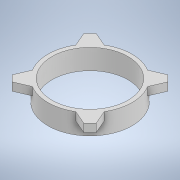
# Autodesk Inventor part: FläktHållare
Saved by Autodesk Inventor 2021 (Build 250183000, 183)
## iProperties
Created: 2025-01-14
Part Number: FläktHållare
Material: Generic
Document SubType Name: Modeling
Designer: 24lucsil
Density: 1 g/cm^3
Appearance: Default
Author: 24lucsil
Autodesk Inventor part; units mm, degrees
ref_plane "YZ Plane" through (0, 0, 0) normal (1, 0, 0) x (0, 1, 0)
ref_plane "XZ Plane" through (0, 0, 0) normal (0, 1, 0) x (-1, 0, 0)
ref_plane "XY Plane" through (0, 0, 0) normal (0, 0, 1) x (1, 0, 0)
sketch "Sketch1" plane through (0, 0, 0) normal (0, 1, 0) x (-1, 0, 0)
  circle A0 centre (0, 0) radius 47
  circle A1 centre (0, 0) radius 52
  line L0 (52, -52) -> (-52, -52) construction
  line L1 (-52, -52) -> (-52, 52) construction
  line L2 (-52, 52) -> (52, 52) construction
  line L3 (52, 52) -> (52, -52) construction
  line L4 (52, -52) -> (52, -44.5) construction
  line L5 (52, -52) -> (44.5, -52) construction
  line L6 (-52, -52) -> (-44.5, -52) construction
  line L7 (-52, -52) -> (-52, -44.5) construction
  line L8 (-52, 52) -> (-44.5, 52) construction
  line L9 (-52, 52) -> (-52, 44.5) construction
  line L10 (52, 52) -> (52, 44.5) construction
  line L11 (52, 52) -> (44.5, 52) construction
  line L12 (52, 52) -> (52, 44.5) construction
  line L13 (52, -44.5) -> (44.5, -52)
  line L14 (-44.5, -52) -> (-52, -44.5)
  line L15 (-52, 44.5) -> (-44.5, 52)
  line L16 (44.5, 52) -> (52, 44.5)
  line L17 (44.5, -52) -> (44.5, -26.9026) construction
  line L18 (52, -44.5) -> (44.5, -26.9026) construction
  line L19 (-44.5, -52) -> (-44.5, -26.9026) construction
  line L20 (-52, -44.5) -> (-44.5, -26.9026) construction
  line L21 (52, -44.5) -> (26.9026, -44.5) construction
  line L22 (44.5, -52) -> (26.9026, -44.5) construction
  line L23 (-52, -44.5) -> (-26.9026, -44.5) construction
  line L24 (-44.5, -52) -> (-26.9026, -44.5) construction
  line L25 (-44.5, 52) -> (-44.5, 26.9026) construction
  line L26 (-52, 44.5) -> (-44.5, 26.9026) construction
  line L27 (-52, 44.5) -> (-26.9026, 44.5) construction
  line L28 (-44.5, 52) -> (-26.9026, 44.5) construction
  line L29 (52, 44.5) -> (26.9026, 44.5) construction
  line L30 (44.5, 52) -> (44.5, 26.9026) construction
  line L31 (44.5, 52) -> (26.9026, 44.5) construction
  line L32 (52, 44.5) -> (44.5, 26.9026) construction
  line L33 (44.5, 52) -> (26.9026, 44.5)
  line L34 (52, 44.5) -> (44.5, 26.9026)
  line L35 (52, -44.5) -> (44.5, -26.9026)
  line L36 (44.5, -52) -> (26.9026, -44.5)
  line L37 (-26.9026, -44.5) -> (-44.5, -52)
  line L38 (-44.5, -26.9026) -> (-52, -44.5)
  line L39 (-44.5, 26.9026) -> (-52, 44.5)
  line L40 (-44.5, 52) -> (-26.9026, 44.5)
  dimension "d1" = 104
  dimension "d0" = 94
  dimension "d6" = 7.5
  dimension "d7" = 7.5
  dimension "d8" = 7.5
  dimension "d9" = 7.5
  dimension "d10" = 7.5
  dimension "d11" = 7.5
  dimension "d12" = 104
  dimension "d13" = 104
  dimension "d15" = 7.5
  dimension "d16" = 7.5
  dimension "d18" = 96.5
  constraints: 82 end point, 10 point on line, 9 perpendicular, 2 coincident, 2 horizontal, 2 vertical, 1 centre point, 1 collinear, 10 other
  measures "d0" diameter of A0
  measures "d6" distance of L0.start L4.end
  measures "d7" distance of L0.start L5.end
  measures "d8" distance of L0.end L6.end
  measures "d9" distance of L9.end L1.end
  measures "d10" distance of L1.end L8.end
  measures "d11" distance of L0.end L7.end
  measures "d12" distance of L1.end L2.end
  measures "d13" distance of L2.end L0.start
  measures "d15" distance from line of L11.end L3
  measures "d16" distance of L10.end L2.end
  measures "d18" distance from line of L37.end L12
extrude "Extrusion1" add sketch "Sketch1" along normal blind 25 contours A1
sketch "Sketch2" plane through (0, 25, 0) normal (0, 1, 0) x (1, 0, 0)
  line L0 (-52, -52) -> (-52, 52) construction
  line L1 (-52, 52) -> (52, 52) construction
  line L2 (52, 52) -> (52, -52) construction
  line L3 (52, -52) -> (-52, -52) construction
  line L4 (-52, -52) -> (-44.5, -52) construction
  line L5 (52, -52) -> (44.5, -52) construction
  line L6 (52, -52) -> (52, -44.5) construction
  line L7 (52, 52) -> (52, 44.5) construction
  line L8 (-52, 52) -> (-52, 44.5) construction
  line L9 (-52, 52) -> (-44.5, 52) construction
  line L10 (52, 52) -> (44.5, 52) construction
  line L11 (52, 44.5) -> (44.5, 52)
  line L12 (-44.5, 52) -> (-52, 44.5)
  line L13 (-44.5, -52) -> (-52, -44.5)
  line L14 (44.5, -52) -> (52, -44.5)
  circle A0 centre (0, 0) radius 52 construction
  line L15 (-52, 44.5) -> (-44.5, 26.9026)
  circle A1 centre (0, 0) radius 52 projected
  line L16 (52, 44.5) -> (44.5, 26.9026)
  line L17 (-44.5, 52) -> (-26.9026, 44.5)
  line L18 (44.5, 52) -> (26.9026, 44.5)
  line L19 (52, -44.5) -> (44.5, -26.9026)
  line L20 (44.5, -52) -> (26.9026, -44.5)
  line L21 (-44.5, -52) -> (-26.9026, -44.5)
  line L22 (-52, -44.5) -> (-44.5, -26.9026)
  dimension "d19" = 104
  dimension "d20" = 104
  dimension "d21" = 52
  dimension "d22" = 52
  dimension "d23" = 7.5
  dimension "d24" = 7.5
  dimension "d25" = 7.5
  dimension "d26" = 7.5
  dimension "d27" = 7.5
  dimension "d28" = 7.5
  dimension "d29" = 7.5
  dimension "d30" = 7.5
  dimension "d31" = 104
  dimension "d32" = 23.084
  dimension "d33" = 156.916
  constraints: 46 end point, 8 point on line, 4 parallel, 4 perpendicular, 2 horizontal, 2 vertical, 1 centre point, 1 coincident, 9 other
  measures "d19" distance between parallel lines of L0 L2
  measures "d20" distance between parallel lines of L1 L3
  measures "d21" distance from line of point (0, 0) L2
  measures "d22" distance from line of point (0, 0) L1
  measures "d23" distance of L4.end L0.start
  measures "d24" distance of L2.end L5.end
  measures "d25" distance of L6.end L2.end
  measures "d26" distance of L1.end L7.end
  measures "d27" distance of L0.end L8.end
  measures "d28" distance of L0.end L9.end
  measures "d29" distance of L1.end L10.end
  measures "d30" distance of L0.start L13.end
  measures "d31" diameter of A0
  measures "d32" angle of L16 L2
  measures "d33" angle of L6 L19
extrude "Extrusion2" add sketch "Sketch2" against normal blind 10 contours L16 A1 L18 L11 | A1 L15 L12 L17 | L19 L14 L20 A1 | A1 L21 L13 L22
body "Solid1"
